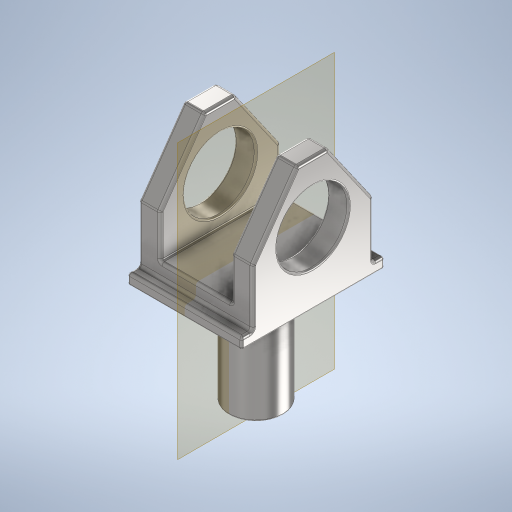
# Autodesk Inventor part: robo_arm_base
Saved by Autodesk Inventor 2023 (Build 270158000, 158)
## iProperties
Created: 2023-11-21
Part Number: robo_arm_base
Material: Steel, Mild
Document SubType Name: Modeling
Designer: Beatrice
Density: 7.85 g/cm^3
Appearance: Semi-Polished
Author: Beatrice
Autodesk Inventor part; units mm, degrees
ref_plane "YZ Plane" through (0, 0, 0) normal (1, 0, 0) x (0, 1, 0)
ref_plane "XZ Plane" through (0, 0, 0) normal (0, 1, 0) x (-1, 0, 0)
sketch "Sketch1" plane through (0, 0, 0) normal (1, 0, 0) x (0, 1, 0)
  line L0 (0, 0) -> (0, 0) construction
  line L1 (10, -10) -> (-10, -10)
  line L2 (-10, -10) -> (-10, 10)
  line L3 (-10, 10) -> (10, 10)
  line L4 (10, 10) -> (10, -10)
  line L5 (10, -10) -> (-10, 10) construction
  line L6 (-10, -10) -> (10, 10) construction
  circle A0 centre (0, 0) radius 5
  line L7 (-10, 0) -> (-2.9979, 10)
  line L8 (-10, 0) -> (2.2077, 0) construction
  line L9 (10, 0) -> (2.9979, 10)
  line L10 (-10, -10) -> (10, -10)
  line L11 (10, -10) -> (10, -6.5)
  line L12 (10, -6.5) -> (-10, -6.5)
  line L13 (-10, -6.5) -> (-10, -10)
  point P0 (-6.499, 5)
  point P1 (6.499, 5)
  dimension "d0" = 20
  dimension "d1" = 10
  dimension "d2" = 20
  dimension "d3" = 55
  dimension "d4" = 3.5
  dimension "d33" = 8.1915
  dimension "d34" = 10
  dimension "d35" = 6.499
  dimension "d36" = 6.499
  dimension "d37" = 55
  dimension "d38" = 10
  dimension "d39" = 70
  constraints: 28 end point, 6 midpoint, 4 parallel, 3 horizontal, 2 coincident, 2 perpendicular, 2 point on line, 1 centre point, 1 equal length, 1 horizontal alignment
  measures "d0" distance of L2.end L3.end
  measures "d1" diameter of A0
  measures "d2" distance of L1.end L2.end
  measures "d3" angle of L8 L7
  measures "d4" distance between parallel lines of L1 L12
  measures "d33" distance from line of point (0, 0) L9
  measures "d34" distance from line of L1 point (0, 0)
  measures "d35" horizontal distance of point (0, 0) point (-6.499, 5)
  measures "d36" horizontal distance of point (0, 0) point (6.499, 5)
  measures "d37" angle of L0 L9
  measures "d38" vertical distance of L9.start L9.end
  measures "d39" angle of L7 L9
extrude "Extrusion1" add sketch "Sketch1" along normal blind 8 contours L1 L2 L12 L4
extrude "Extrusion2" add sketch "Sketch1" along normal blind 3 contours L12 L2 L7 L3 L9 L4
ref_plane "Work Plane1" through (8, 0, 0) normal (1, 0, 0) x (0, 0, -1)
mirror "Mirror1" about plane through (8, 0, 0) normal (1, 0, 0) of "Extrusion2", "Extrusion1"
sketch "Sketch2" plane through (0, -10, -10) normal (0, 0, -1) x (-1, 0, 0)
  line L0 (22, 0) -> (0, 0) construction
  arc A0 (22, 0) -> (22.5, 0.5) centre (22, 0.5) ccw construction
  line L1 (22.5, 17.5) -> (22.5, 0.5) construction
  arc A1 (22.5, 17.5) -> (22, 18) centre (22, 17.5) ccw construction
  line L2 (0, 18) -> (22, 18) construction
  arc A2 (0, 18) -> (-0.5, 17.5) centre (0, 17.5) ccw construction
  line L3 (-0.5, 0.5) -> (-0.5, 17.5) construction
  arc A3 (-0.5, 0.5) -> (0, 0) centre (0, 0.5) ccw construction
  line L4 (-4.5, 10) -> (-11.5, 10) construction
  circle A4 centre (13, 10) radius 7.5
  circle A5 centre (13, 10) radius 8.4
  circle A6 centre (13, 10) radius 8.9443
  line L5 (0, 0) -> (0, 20) projected
  line L6 (0, 20) -> (-16, 20) projected
  line L7 (-16, 0) -> (-16, 20) projected
  line L8 (0, 0) -> (-16, 0) projected
  line L9 (-3, 0) -> (-13, 0) projected
  line L10 (-8, 0) -> (-8, 20)
  line L11 (-3, 20) -> (-13, 20) projected
  line L12 (0, 10) -> (-16, 10)
  circle A7 centre (-8, 10) radius 3.8
  circle A8 centre (-8, 10) radius 4.7
  circle A9 centre (-8, 10) radius 5.7
  point P0 (23.5, 9)
  point P1 (-11.5, 10)
  point P2 (-3.3, 10)
  point P3 (-12.7, 10)
  dimension "d10" = 15
  dimension "d11" = 0.9
  dimension "d12" = 17.8885
  dimension "d13" = 7.6
  dimension "d14" = 0.9
  dimension "d28" = 1
  constraints: 12 end point, 10 centre point, 8 point on circle, 4 midpoint, 1 coincident, 5 other
  measures "d10" diameter of A4
  measures "d11" radial gap between concentric circles of A4 A5
  measures "d12" diameter of A6
  measures "d13" diameter of A7
  measures "d14" radial gap between concentric circles of A7 A8
  measures "d28" radial gap between concentric circles of A8 A9
extrude "Extrusion3" add sketch "Sketch2" along normal blind 15 contours A7 L10 L12 | L12 L10 A7 | L12 A7 L10 | L10 A7 L12
fillet "Fillet1" radius 0.25 33 edges at (3, -6.499, 5) (0, -6.499, 5) (0, 0, 10) (3, 0, 10) (3, 6.499, 5) (0, 6.499, 5) (3, 10, -3.25) (0, 10, -5) (3, -10, -3.25) (0, -10, -5) (13, -10, -3.25) (16, -10, -5) (16, -6.499, 5) (13, -6.499, 5) (13, 0, 10) (16, 0, 10) (16, 6.499, 5) (13, 6.499, 5) (16, 10, -5) (13, 10, -3.25) (8, 10, -6.5) (8, 10, -10) (16, 0, -10) (8, -10, -10) (8, -10, -6.5) (3, 0, -6.5) (13, 0, -6.5) (13, -5, 0) (16, -5, 0) (0, -5, 0) (3, -5, 0) (0, 0, -10) (11.8, 0, -10)
fillet "Fillet2" radius 0.25 1 edges at (11.8, 0, -25)
fillet "Fillet3" radius 2 24 edges at (2.9268, -9.9268, -0.0231) (0.0732, -9.9268, -0.0231) (14.5, -10, 0) (1.5, -10, 0) (2.9268, -2.9598, 9.9268) (0.0732, -2.9598, 9.9268) (1.5, -2.9979, 10) (2.9268, 2.9598, 9.9268) (0.0732, 2.9598, 9.9268) (1.5, 2.9979, 10) (13.0732, -9.9268, -0.0231) (15.9268, -9.9268, -0.0231) (13.0732, -2.9598, 9.9268) (15.9268, -2.9598, 9.9268) (14.5, -2.9979, 10) (13.0732, 2.9598, 9.9268) (15.9268, 2.9598, 9.9268) (14.5, 2.9979, 10) (2.9268, 9.9268, -0.0231) (0.0732, 9.9268, -0.0231) (14.5, 10, 0) (1.5, 10, 0) (13.0732, 9.9268, -0.0231) (15.9268, 9.9268, -0.0231)
extrude "Extrusion5" add sketch "Sketch2" along normal blind 1 contours A9 L10 A8 L12 | L12 A8 L10 A9 | L10 A8 L12 A9 | A9 L12 A8 L10
fillet "Fillet4" radius 0.4 3 edges at (13.7, 0, -11) (12.7, 0, -11) (12.7, 0, -10)
ref_plane "Work Plane3" through (8, -9.75, -9.75) normal (1, 0, 0) x (0, 0, -1)
sketch "Sketch4" plane through (0, 0, 0) normal (-1, 0, 0) x (0, 0, 1)
  arc A0 (0.3732, 9.4335) -> (-0.6306, 9.75) centre (-0.6306, 8) ccw projected
  line L0 (-9.75, 9.75) -> (-0.6306, 9.75) projected
  line L1 (-9.75, -9.75) -> (-9.75, 9.75) projected
  line L2 (-0.6306, -9.75) -> (-9.75, -9.75) projected
  arc A1 (-0.6306, -9.75) -> (0.3732, -9.4335) centre (-0.6306, -8) ccw projected
  line L3 (9.0038, -3.3903) -> (0.3732, -9.4335) projected
  arc A2 (9.0038, -3.3903) -> (9.75, -1.9568) centre (8, -1.9568) ccw projected
  line L4 (9.75, 1.9568) -> (9.75, -1.9568) projected
  arc A3 (9.75, 1.9568) -> (9.0038, 3.3903) centre (8, 1.9568) ccw projected
  line L5 (0.3732, 9.4335) -> (9.0038, 3.3903) projected
  circle A4 centre (0, 0) radius 5.25 projected
  arc A5 (8.4441, 1.9568) -> (8.2547, 2.3206) centre (8, 1.9568) ccw
  line L6 (8.4441, 1.9568) -> (8.4441, -1.9568)
  arc A6 (8.2547, -2.3206) -> (8.4441, -1.9568) centre (8, -1.9568) ccw
  line L7 (8.2547, -2.3206) -> (-0.3759, -8.3638)
  arc A7 (-0.6306, -8.4441) -> (-0.3759, -8.3638) centre (-0.6306, -8) ccw
  line L8 (-0.6306, -8.4441) -> (-8.4441, -8.4441)
  line L9 (-8.4441, -12.6223) -> (-8.4441, 12.6223)
  line L10 (-8.4441, 8.4441) -> (-0.6306, 8.4441)
  arc A8 (-0.3759, 8.3638) -> (-0.6306, 8.4441) centre (-0.6306, 8) ccw
  line L11 (-0.3759, 8.3638) -> (8.2547, 2.3206)
  arc A9 (12.6223, 1.9568) -> (10.6512, 5.7432) centre (8, 1.9568) ccw
  line L12 (12.6223, 1.9568) -> (12.6223, -1.9568)
  arc A10 (10.6512, -5.7432) -> (12.6223, -1.9568) centre (8, -1.9568) ccw
  line L13 (10.6512, -5.7432) -> (2.0206, -11.7864)
  arc A11 (-0.6306, -12.6223) -> (2.0206, -11.7864) centre (-0.6306, -8) ccw
  line L14 (-0.6306, -12.6223) -> (-12.6223, -12.6223)
  line L15 (-12.6223, -12.6223) -> (-12.6223, 12.6223)
  line L16 (-12.6223, 12.6223) -> (-0.6306, 12.6223)
  arc A12 (2.0206, 11.7864) -> (-0.6306, 12.6223) centre (-0.6306, 8) ccw
  line L17 (2.0206, 11.7864) -> (10.6512, 5.7432)
  constraints: 24 end point, 16 point on circle, 8 centre point, 4 point on line, 14 other
extrude "Extrusion6" cut sketch "Sketch4" against normal through all contours L5 A3 L4 A2 L3 A1 L2 L9 L8 A7 L7 A6 L6 A5 L11 A8 L10 L0 A0 | A0 L0 L9 L16 A12 L17 A9 L12 A10 L13 A11 L14 L2 A1 L3 A2 L4 A3 L5
fillet "Fillet5" radius 0.4 54 edges at (0, 8.4236, -0.497) (0, 8.4441, -4.5374) (0, 2.1619, 8.3939) (0, 0, 8.4441) (0, -2.1619, 8.3939) (0, -5.3422, 3.9394) (0, -8.4236, -0.497) (0, -8.4441, -4.5374) (0, 5.3422, 3.9394) (16, 8.4236, -0.497) (16, 5.3422, 3.9394) (16, 2.1619, 8.3939) (16, 0, 8.4441) (16, -2.1619, 8.3939) (16, -5.3422, 3.9394) (16, -8.4236, -0.497) (16, -8.4441, -4.5374) (16, 8.4441, -4.5374) (12.9268, 8.4441, -6.4268) (8, 8.4441, -6.5) (3.0732, 8.4441, -6.4268) (3, 8.4441, -3.4403) (3, 8.4236, -0.497) (3, 5.3422, 3.9394) (3, 2.1619, 8.3939) (3, 0, 8.4441) (3, -2.1619, 8.3939) (3, -5.3422, 3.9394) (3, -8.4236, -0.497) (3, -8.4441, -3.4403) (3.0732, -8.4441, -6.4268) (8, -8.4441, -6.5) (12.9268, -8.4441, -6.4268) (13, -8.4441, -3.4403) (13, -8.4236, -0.497) (13, -5.3422, 3.9394) (13, -2.1619, 8.3939) (13, 0, 8.4441) (13, 2.1619, 8.3939) (13, 5.3422, 3.9394) (13, 8.4236, -0.497) (13, 8.4441, -3.4403) (8, 8.4441, -8.4441) (15.9268, 9.9268, -8.4441) (16, 9.0971, -8.4441) (0.0732, 9.9268, -8.4441) (0, 9.0971, -8.4441) (8, 10, -8.4441) (0.0732, -9.9268, -8.4441) (8, -10, -8.4441) (15.9268, -9.9268, -8.4441) (16, -9.0971, -8.4441) (0, -9.0971, -8.4441) (8, -8.4441, -8.4441)
body "Solid1"
